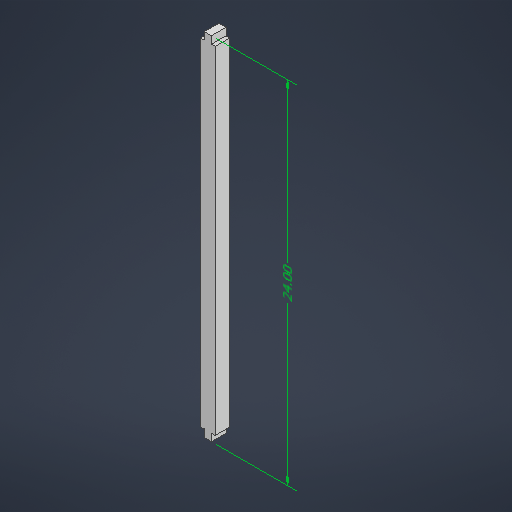
# Autodesk Inventor part: pieza individual
Saved by Autodesk Inventor 2027 (Build 310192000, 192)
## iProperties
Created: 2026-04-14
Part Number: pieza individual
Material: Genérico
Document SubType Name: Modeling
Designer: leand
Density: 1 g/cm^3
Appearance: Valor por defecto
Author: leand
Autodesk Inventor part; units mm, degrees
ref_plane "YZ Plane" through (0, 0, 0) normal (1, 0, 0) x (0, 1, 0)
ref_plane "XZ Plane" through (0, 0, 0) normal (0, 1, 0) x (-1, 0, 0)
ref_plane "XY Plane" through (0, 0, 0) normal (0, 0, 1) x (1, 0, 0)
sketch "Boceto1" plane through (0, 0, 0) normal (0, 0, 1) x (1, 0, 0)
  line L0 (6.7952, 10.0888) -> (6.7952, -12.4112)
  line L1 (7.0459, 11.0888) -> (7.5344, 11.0888)
  line L2 (7.0459, -12.4112) -> (7.0459, -12.9112)
  line L3 (7.5344, -12.4112) -> (7.5344, -12.9112)
  line L4 (7.5344, -12.9112) -> (7.0459, -12.9112)
  line L5 (6.7952, -12.4112) -> (7.0459, -12.4112)
  line L6 (7.5344, -12.4112) -> (7.7952, -12.4112)
  line L7 (6.7952, 10.0888) -> (6.7952, 10.5888)
  line L8 (7.0459, 11.0888) -> (7.5344, 11.0888)
  line L9 (7.5344, 11.0888) -> (7.5344, 10.5888)
  line L10 (7.0459, 11.0888) -> (7.0459, 10.5888)
  line L11 (6.7952, 10.5888) -> (7.0459, 10.5888)
  line L12 (7.5344, 10.5888) -> (7.7952, 10.5888)
  line L13 (7.7952, 10.5888) -> (7.7952, -12.4112)
  point P0 (0, 0)
  constraints: 28 end point, 4 perpendicular, 3 vertical, 1 horizontal
extrude "Extrusión1" add sketch "Boceto1" along normal mid plane 1
